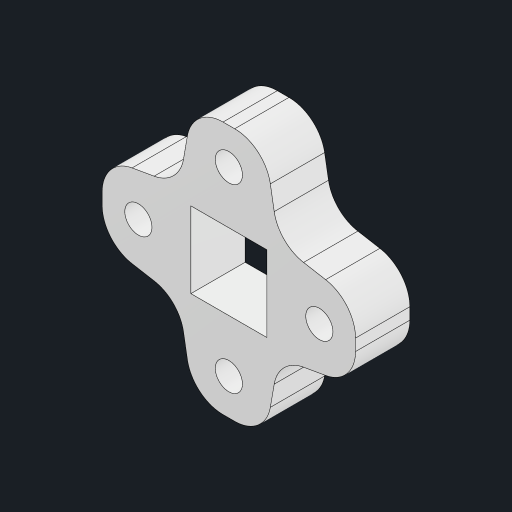
# Autodesk Inventor part: WireHolder
Saved by Autodesk Inventor 2023 (Build 270158000, 158)
## iProperties
Created: 2022-06-04
Part Number: WireHolder
Material: ABS プラスチック
Document SubType Name: Modeling
Designer: neko2
Density: 1.06 g/cm^3
Appearance: 滑らか - 白
Mass: 0.272855 g
Surface Area: 3.71056 cm^2
Volume: 0.257411 cm^3
Author: neko2
Autodesk Inventor part; units mm, degrees
ref_plane "YZ Plane" through (0, 0, 0) normal (1, 0, 0) x (0, 1, 0)
ref_plane "XZ Plane" through (0, 0, 0) normal (0, 1, 0) x (-1, 0, 0)
ref_plane "XY Plane" through (0, 0, 0) normal (0, 0, 1) x (1, 0, 0)
sketch "スケッチ1" plane through (0, 0, 0) normal (0, 0, 1) x (1, 0, 0)
  line L0 (2, 7) -> (-2, 7)
  line L1 (-2, 7) -> (-2.7495, 2.7495)
  circle A0 centre (0, 5) radius 0.75
  line L2 (0, 0) -> (-4.3694, 4.3694)
  line L3 (0, 0) -> (4.0735, 4.0735)
  line L4 (2, 7) -> (2.7495, 2.7495)
  line L5 (-7, -2) -> (-2.7495, -2.7495)
  line L6 (-7, 2) -> (-7, -2)
  line L7 (-7, 2) -> (-2.7495, 2.7495)
  circle A1 centre (-5, 0) radius 0.75
  line L8 (2, -7) -> (2.7495, -2.7495)
  line L9 (-2, -7) -> (2, -7)
  line L10 (-2, -7) -> (-2.7495, -2.7495)
  circle A2 centre (0, -5) radius 0.75
  line L11 (7, 2) -> (2.7495, 2.7495)
  line L12 (7, -2) -> (7, 2)
  line L13 (7, -2) -> (2.7495, -2.7495)
  circle A3 centre (5, 0) radius 0.75
  line L14 (2.1, 2.1) -> (-2.1, 2.1)
  line L15 (-2.1, 2.1) -> (-2.1, -2.1)
  line L16 (-2.1, -2.1) -> (2.1, -2.1)
  line L17 (2.1, -2.1) -> (2.1, 2.1)
  line L18 (0, 5) -> (5, 0)
  point P0 (0, 7)
  point P1 (-7, 0)
  point P2 (0, -7)
  point P3 (7, 0)
  point P4 (-2.7495, -2.7495)
  point P5 (2.7495, 2.7495)
  point P6 (-2.1, 0)
  point P7 (0, 2.1)
  dimension "d12" = 4
  dimension "d13" = 1.5
  dimension "d15" = 5
  dimension "d19" = 2
  dimension "d22" = 90
  dimension "d23" = 100
  dimension "d26" = 360
  dimension "d28" = 4.2
  constraints: 38 end point, 4 centre point, 3 midpoint, 3 vertical alignment, 2 coincident, 2 equal length, 2 horizontal, 2 horizontal alignment, 2 parallel, 2 point on line, 1 perpendicular, 41 other
  measures "d12" distance of L0.start L0.end
  measures "d13" diameter of A0
  measures "d15" distance of point (0, 0) L18.start
  measures "d19" distance of point (0, 7) L18.start
  measures "d22" angle of L3 L2
  measures "d23" angle of L0 L1
  measures "d28" distance of L14.end L15.end
extrude "押し出し1" add sketch "スケッチ1" along normal blind 3 contours L4 L3 L14 L2 L1 L0 | L11 L12 L13 L8 L9 L10 L5 L6 L7 L2 L15 L16 L17 L3
fillet "フィレット1" radius 2 12 edges at (2, 7, 1.5) (-2, 7, 1.5) (-7, 2, 1.5) (-7, -2, 1.5) (-2, -7, 1.5) (-2.7495, -2.7495, 1.5) (-2.7495, 2.7495, 1.5) (2.7495, 2.7495, 1.5) (7, 2, 1.5) (7, -2, 1.5) (2.7495, -2.7495, 1.5) (2, -7, 1.5)
